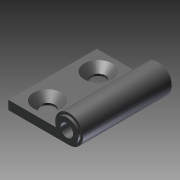
# Autodesk Inventor part: HHPFLN5-2
Saved by Autodesk Inventor 2011 SP1 (Build 150282100, 282)
## iProperties
Created: 2015-01-26
Part Number: HHPFLN5-2
Catalog Web Link: www.cadenas.de
Description: HHPFLN, HHPFRN-2-Aluminum Flag Hinges
Vendor: MISUMI
Document SubType Name: Modeling
Designer: PARTuser1
Manufacturer: MISUMI
Mass: 4.86234 g
Surface Area: 35.1362 cm^2
Volume: 4.86234 cm^3
Density: 1 g/cm^3
Category: PARTsolutions
Company: MISUMI
Title: HHPFLN5-2
Author: Cadenas PARTsolutions
Comments: Aluminum Flag Hinges
PSOL_IDENT_0: {\\10.0.0.236\data_v8\23d-libs\misumi\metric\39_accessories_for_al_extrusions\hhpfln_2.prj},177 {VTY
PSOL_IDENT_1: P=3D},{NB=HHPFLN5-2},{LINA=HHPFLN5-2},{NN=HHPFLN, HHPFRN-2},{DATE=17.11.2014 05:31:02},{GEOMDATE=07.
PSOL_IDENT_2: 05.2009 08:36:00},{VERSION=},{LINEID=10},{LINESUBID=-1},{WBVAR=TS,ALT1}  {NB=HHPFLN5-2},{LINA=HHPFLN
PSOL_IDENT_3: 5-2},{KT=DUMMY},{PN=HHPFLN5},{TYPE=HHPFLN},{TS=HHPFLN},{MAT=6063 Aluminum Bushing - Polyacetal},{ST=
PSOL_IDENT_4: Anodizing},{NO=5},{ALKG=10},{ALN=98},{MASS=36},{L=35},{W=48},{K=7.5},{P=20},{J=8.0},{F=16.0},{V=10.5
PSOL_IDENT_5: },{ND=5.5},{NC=11},{T=3.5},{Y=38.5},{AB=FB5-8},{QB=4},{AN=HNTT5-5},{QN=4},{ALT1=}
SUPPLIER: MISUMI
ARTICLENO: HHPFLN5-2
BOMINFO: HHPFLN5-2
CREATOR: CADENAS GmbH
Autodesk Inventor part; units mm, degrees
ref_plane "YZ Plane" through (0, 0, 0) normal (1, 0, 0) x (0, 1, 0)
ref_plane "XZ Plane" through (0, 0, 0) normal (0, 1, 0) x (-1, 0, 0)
ref_plane "XY Plane" through (0, 0, 0) normal (0, 0, 1) x (1, 0, 0)
sketch "Sketch_1" plane through (0, 0, 0) normal (0, 0, 1) x (1, 0, 0)
  line L0 (0, 0) -> (0, 36.8)
  line L1 (0, 36.8) -> (4.5, 36.8)
  line L2 (4.5, 36.8) -> (4.5, 35.9)
  line L3 (4.5, 35.9) -> (5.5, 35.9)
  line L4 (5.5, 35.9) -> (5.5, 0.9)
  line L5 (5.5, 0.9) -> (4.5, 0.9)
  line L6 (4.5, 0.9) -> (4.5, 0)
  line L7 (4.5, 0) -> (0, 0)
  line L8 (0, 0) -> (0, 36.8)
  constraints: 18 end point
revolve "Revolution1" add sketch "Sketch_1" angle 360 about axis through (0, 0, 0) along (0, -1, 0)
sketch "Sketch_2" plane through (0, 0, -5.5) normal (0, 0, 1) x (1, 0, 0)
  line L0 (-24, 0.9) -> (0, 0.9)
  line L1 (0, 0.9) -> (0, 35.9)
  line L2 (0, 35.9) -> (-24, 35.9)
  line L3 (-24, 35.9) -> (-24, 0.9)
  constraints: 8 end point
extrude "Extrusion1" add sketch "Sketch_2" along normal blind 3.5
sketch "Sketch_4" plane through (-16, 0, 0) normal (1, 0, 0) x (0, 0, -1)
  line L0 (2, 8.4) -> (5.5, 8.4)
  line L1 (5.5, 8.4) -> (5.5, 5.65)
  line L2 (5.5, 5.65) -> (4.75, 5.65)
  line L3 (4.75, 5.65) -> (2, 2.9)
  line L4 (2, 2.9) -> (2, 8.4)
  line L5 (2, 8.4) -> (5.5, 8.4)
  constraints: 12 end point
revolve "Revolution2" cut sketch "Sketch_4" angle 360 about axis through (-16, 8.4, -2) along (0, 0, 1)
sketch "Sketch_5" plane through (-16, 0, 0) normal (1, 0, 0) x (0, 0, -1)
  line L0 (2, 28.4) -> (5.5, 28.4)
  line L1 (5.5, 28.4) -> (5.5, 25.65)
  line L2 (5.5, 25.65) -> (4.75, 25.65)
  line L3 (4.75, 25.65) -> (2, 22.9)
  line L4 (2, 22.9) -> (2, 28.4)
  line L5 (2, 28.4) -> (5.5, 28.4)
  constraints: 12 end point
revolve "Revolution3" cut sketch "Sketch_5" angle 360 about axis through (-16, 28.4, -2) along (0, 0, 1)
sketch "Sketch_9" plane through (0, 0, 0) normal (0, 0, 1) x (1, 0, 0)
  line L0 (0, 0) -> (0, 36.8)
  line L1 (0, 36.8) -> (2.5, 36.8)
  line L2 (2.5, 36.8) -> (2.5, 0)
  line L3 (2.5, 0) -> (0, 0)
  line L4 (0, 0) -> (0, 36.8)
  constraints: 10 end point
revolve "Revolution4" cut sketch "Sketch_9" angle 360 about axis through (0, 0, 0) along (0, -1, 0)
ref_plane "2_XY" through (0, 0, 0) normal (0, 1, 0) x (1, 0, 0)
ref_plane "2_YZ" through (0, 0, 0) normal (1, 0, 0) x (0, 0, -1)
ref_plane "2_ZX" through (0, 0, 0) normal (0, 0, -1) x (0, 1, 0)
ref_plane "to_bolt3_r_XY" through (16, 28.4, -2) normal (0, 0, 1) x (1, 0, 0)
ref_plane "to_bolt3_r_YZ" through (16, 28.4, -2) normal (1, 0, 0) x (0, 1, 0)
ref_plane "to_bolt3_r_ZX" through (16, 28.4, -2) normal (0, 1, 0) x (0, 0, 1)
ref_plane "to_bolt4_r_XY" through (16, 8.4, -2) normal (0, 0, 1) x (1, 0, 0)
ref_plane "to_bolt4_r_YZ" through (16, 8.4, -2) normal (1, 0, 0) x (0, 1, 0)
ref_plane "to_bolt4_r_ZX" through (16, 8.4, -2) normal (0, 1, 0) x (0, 0, 1)
ref_plane "to_bolt3_XY" through (-16, 28.4, -2) normal (0, 0, 1) x (1, 0, 0)
ref_plane "to_bolt3_YZ" through (-16, 28.4, -2) normal (1, 0, 0) x (0, 1, 0)
ref_plane "to_bolt3_ZX" through (-16, 28.4, -2) normal (0, 1, 0) x (0, 0, 1)
ref_plane "to_bolt4_XY" through (-16, 8.4, -2) normal (0, 0, 1) x (1, 0, 0)
ref_plane "to_bolt4_YZ" through (-16, 8.4, -2) normal (1, 0, 0) x (0, 1, 0)
ref_plane "to_bolt4_ZX" through (-16, 8.4, -2) normal (0, 1, 0) x (0, 0, 1)
body "Solid1"
